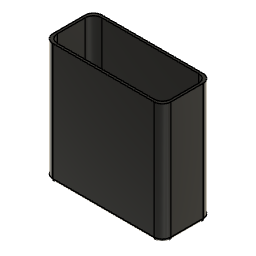
Wireless sensor holder (Autodesk Fusion 360 design; units mm, degrees)
Autodesk Fusion 360 part; units mm, degrees
sketch "Sketch1" plane through (0, 0, 0) normal (0, 0, 1) x (1, 0, 0)
  line L0 (0, 0) -> (25.5, 0)
  line L1 (25.5, 0) -> (25.5, -10.6)
  line L2 (25.5, -10.6) -> (0, -10.6)
  line L3 (0, -10.6) -> (0, 0)
  dimension "d1" = 10.6
  dimension "d2" = 25.5
  constraint horizontal L0
  constraint vertical L1
  constraint horizontal L2
  constraint vertical L3
  constraint coincident L0.start L3.end
  measures "d1" distance of L0.end L1.end
  measures "d2" distance of L1.end L2.end
extrude "Extrude1" add sketch "Sketch1" along normal blind 1
sketch "Sketch2" plane through (0, 0, 1) normal (0, 0, 1) x (-1, 0, 0)
  line L0 (0, 10.6) -> (-25.5, 10.6)
  line L1 (-25.5, 10.6) -> (-25.5, 0)
  line L2 (-25.5, 0) -> (0, 0)
  line L3 (0, 0) -> (0, 10.6)
  line L4 (-0.5, 0.5) -> (-25, 0.5)
  line L5 (-25, 0.5) -> (-25, 10.1)
  line L6 (-25, 10.1) -> (-0.5, 10.1)
  line L7 (-0.5, 10.1) -> (-0.5, 0.5)
  line L8 (-25.5, 10.6) -> (0, 10.6)
  dimension "d5" = 0.5
  dimension "d6" = 0.5
  dimension "d26" = 0.5
  dimension "d27" = 0.5
  constraint horizontal L4
  constraint vertical L5
  constraint horizontal L6
  constraint vertical L7
  measures "d5" distance of L3 L7
  measures "d6" distance of L6 L8
  measures "d26" distance of L1 L5
  measures "d27" distance of L2 L4
extrude "Extrude2" add sketch "Sketch2" along normal blind 25
sketch "Sketch3" plane through (0, 0, 0) normal (0, 0, -1) x (1, 0, 0)
  line L0 (25.5, 10.6) -> (0, 10.6)
  line L1 (0, 10.6) -> (0, 0)
  line L2 (0, 0) -> (25.5, 0)
  line L3 (25.5, 0) -> (25.5, 10.6)
  line L4 (7.25, 8.3) -> (18.25, 8.3)
  line L5 (18.25, 8.3) -> (18.25, 2.3)
  line L6 (18.25, 2.3) -> (7.25, 2.3)
  line L7 (7.25, 2.3) -> (7.25, 8.3)
  dimension "d12" = 11
  dimension "d13" = 6
  dimension "d14" = 2.3
  dimension "d15" = 7.25
  dimension "d28" = 25.5
  dimension "d29" = 10.6
  constraint horizontal L4
  constraint vertical L5
  constraint horizontal L6
  constraint vertical L7
  measures "d12" distance of L5.end L6.end
  measures "d13" distance of L4.end L5.end
  measures "d14" distance of L0 L4
  measures "d15" distance of L1 L7
  measures "d28" distance of L0.start L0.end
  measures "d29" distance of L0.start L2.end
extrude "Extrude3" cut sketch "Sketch3" against normal blind 11 contours L4 L5 L6 L7
fillet "Fillet1" radius 1.8 4 edges at (25, -10.1, 13.5) (0.5, -0.5, 13.5) (0.5, -10.1, 13.5) (25, -0.5, 13.5)
fillet "Fillet2" radius 1.8 4 edges at (0, -10.6, 13) (25.5, -10.6, 13) (25.5, 0, 13) (0, 0, 13)
fillet "Fillet3" radius 0.7 8 edges at (0.5272, -10.0728, 0) (0, -5.3, 0) (0.5272, -0.5272, 0) (12.75, 0, 0) (24.9728, -0.5272, 0) (25.5, -5.3, 0) (24.9728, -10.0728, 0) (12.75, -10.6, 0)
equation "d14 = ( d29 - d13 ) / 2"
equation "d15 = ( d28 - d12 ) / 2"
